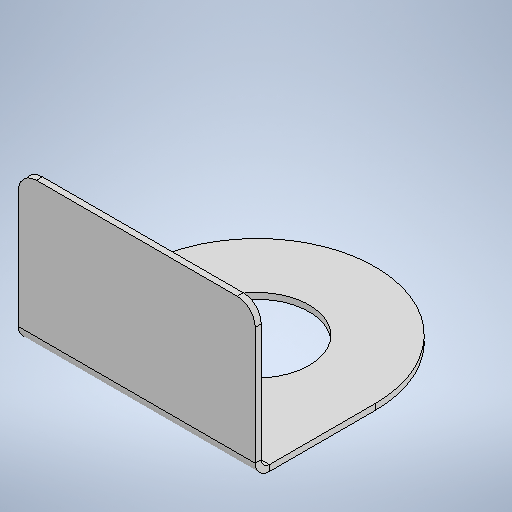
# Autodesk Inventor part: D-ring 11
Saved by Autodesk Inventor 2025.1 (Build 291241020, 241B)
## iProperties
Created: 2024-11-05
Part Number: D-ring 11
Material: Stainless Steel
Document SubType Name: Sheet Metal
Designer: user
Density: 8 g/cm^3
Sheet Metal Rule: AISI304 2mm Die16
Sheet Metal Width: 79.000 mm
Sheet Metal Length: 125.702 mm
Sheet Metal Area: 9930.457 mm^2
Appearance: Default
Flat Pattern Width: 7.9 cm
Flat Pattern Length: 12.5702 cm
Flat Pattern Area: 99.3046 cm^2
Author: user
Autodesk Inventor part; units mm, degrees
ref_plane "YZ Plane" through (0, 0, 0) normal (1, 0, 0) x (0, 1, 0)
ref_plane "XZ Plane" through (0, 0, 0) normal (0, 1, 0) x (-1, 0, 0)
ref_plane "XY Plane" through (0, 0, 0) normal (0, 0, 1) x (1, 0, 0)
sketch "Sketch1" plane through (0, 0, 0) normal (0, 0, 1) x (1, 0, 0)
  line L0 (-39.5, 0) -> (39.5, 0)
  line L1 (-39.5, 0) -> (-39.5, 40)
  arc A0 (39.5, 40) -> (-39.5, 40) centre (0, 40) ccw
  line L2 (39.5, 40) -> (39.5, 0)
  circle A1 centre (0, 40) radius 17.5
  point P0 (0, 0)
  point P1 (0, 0)
  dimension "d6" = 35
  dimension "d7" = 22
  dimension "d8" = 40
  measures "d6" diameter of A1
  measures "d7" radial gap between concentric circles of A1 A0
  measures "d8" distance from line of L0 A0.centre
extrude "Plate1" add sketch "Sketch1" along normal blind 2
sketch "Sketch3" plane through (39.5, 2, 0) normal (0, -1, 0) x (1, 0, 0)
  line L0 (-79, 0) -> (0, 0)
  line L1 (0, 0) -> (0, 50)
  line L2 (0, 50) -> (-79, 50)
  line L3 (-79, 50) -> (-79, 0)
  constraints: 6 end point, 1 horizontal, 1 perpendicular, 1 vertical
edge flange "Flange1" height 50 angle 90 thickness 2 bend radius 2.75 thickness toward (0, -1, 0) relief round relief width 2 relief depth 1 edges at (0, 0, 2) wall of the first edge with corners at (-39.5, 2, 0) (39.5, 2, 0) (39.5, 2, 50) (-39.5, 2, 50)
bend "Bend1"
corner "Corner1"
fillet "Corner Round1" radius 6 2 edges at (39.5, 1, 50) (-39.5, 1, 50)
equation "\"d2\" = Thickness"
equation "\"d9\" = BendReliefWidth"
equation "\"d10\" = BendReliefDepth"
equation "\"d11\" = MinimumRemnant"
equation "\"d12\" = TransitionRadius"
equation "\"d15\" = BendRadius"
equation "\"d16\" = CornerReliefSize"
equation "\"d17\" = GapSize"
equation "\"d18\" = JacobiRadiusSize"
equation "\"BendReliefWidth\" = Thickness"
equation "\"BendReliefDepth\" = 0.5 * Thickness"
equation "\"CornerReliefSize\" = 4 * Thickness"
equation "\"MinimumRemnant\" = 2 * Thickness"
equation "\"TransitionRadius\" = BendRadius"
equation "\"JacobiRadiusSize\" = BendRadius"
equation "\"GapSize\" = Thickness"
equation "\"Thickness\" = 2"
equation "\"BendRadius\" = 2.75"
body "Solid1"
